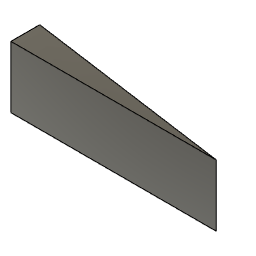
StepenicaZaKosuRavanZaGol v1 (Autodesk Fusion 360 design; units mm, degrees)
Autodesk Fusion 360 part; units mm, degrees
sketch "Sketch1" plane through (0, 0, 0) normal (0, 0, 1) x (1, 0, 0)
  line L0 (25, 25) -> (25, 32)
  line L1 (25, 32) -> (74.9141, 25)
  line L2 (74.9141, 25) -> (25, 25)
  dimension "d1" = 7
  constraint vertical L0
  constraint perpendicular L0 L2
  measures "d1" distance of L0.start L0.end
extrude "Extrude1" add sketch "Sketch1" along normal blind 15
